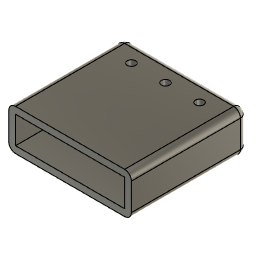
Hülle (Autodesk Fusion 360 design; units mm, degrees)
Autodesk Fusion 360 part; units mm, degrees
sketch "Skizze1" plane through (0, 0, 0) normal (0, 0, 1) x (1, 0, 0)
  line L0 (-50, 50) -> (40, 50)
  line L1 (40, 50) -> (40, -35)
  line L2 (40, -35) -> (-50, -35)
  line L3 (-50, -35) -> (-50, 50)
  dimension "d1" = 90
  dimension "d2" = 85
  constraint horizontal L0
  constraint vertical L1
  constraint horizontal L2
  constraint vertical L3
  measures "d1" distance of L0.start L0.end
  measures "d2" distance of L0.start L2.end
extrude "Extrusion1" add sketch "Skizze1" along normal blind 30
shell "Schale1" thickness 5 removed faces 1 at (10, -35, 20)
fillet "Abrundung1" radius 5 1 edges at (-5, 50, 30)
fillet "Abrundung2" radius 5 3 edges at (40, 5, 30) (40, 48.5355, 28.5355) (40, 50, 12.5)
fillet "Abrundung3" radius 5 3 edges at (-50, 50, 12.5) (-50, 48.5355, 28.5355) (-50, 5, 30)
fillet "Abrundung4" radius 5 5 edges at (-50, 5, 0) (-48.5355, 48.5355, 0) (-5, 50, 0) (38.5355, 48.5355, 0) (40, 5, 0)
sketch "Skizze2" plane through (0, 0, 30) normal (0, 0, 1) x (-1, 0, 0)
  line L0 (45, -45) -> (45, 35)
  line L1 (45, 35) -> (-35, 35)
  line L2 (-35, 35) -> (-35, -45)
  line L3 (-35, -45) -> (45, -45)
  circle A0 centre (5, -35) radius 3
  circle A1 centre (30, -35) radius 3
  circle A2 centre (-20, -35) radius 3
extrude "Extrusion2" cut sketch "Skizze2" along normal mid plane 10 contours A1
extrude "Extrusion3" cut sketch "Skizze2" along normal mid plane 10 contours A0 | A2
